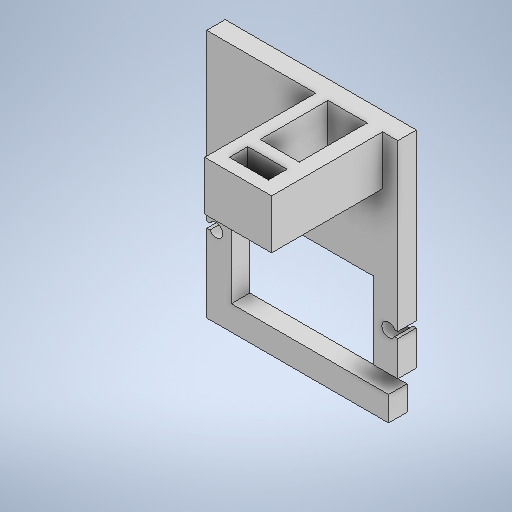
# Autodesk Inventor part: SoporteServo v2
Saved by Autodesk Inventor 2025.2 (Build 292293000, 293)
## iProperties
Created: 2025-05-14
Part Number: SoporteServo v2
Material: Generic
Document SubType Name: Modeling
Designer: cdavi
Density: 1 g/cm^3
Appearance: Default
Author: cdavi
Autodesk Inventor part; units mm, degrees
ref_plane "YZ Plane" through (0, 0, 0) normal (1, 0, 0) x (0, 1, 0)
ref_plane "XZ Plane" through (0, 0, 0) normal (0, 1, 0) x (-1, 0, 0)
ref_plane "XY Plane" through (0, 0, 0) normal (0, 0, 1) x (1, 0, 0)
sketch "Sketch1" plane through (0, 0, 0) normal (0, 0, 1) x (1, 0, 0)
  line L0 (-11.35, -6.15) -> (11.35, -6.15) construction
  line L1 (11.35, -6.15) -> (11.35, 6.15) construction
  line L2 (11.35, 6.15) -> (-11.35, 6.15) construction
  line L3 (-11.35, 6.15) -> (-11.35, -6.15) construction
  line L4 (-11.35, -6.15) -> (11.35, 6.15) construction
  line L5 (11.35, -6.15) -> (-11.35, 6.15) construction
  line L6 (-11.5, -6.3) -> (11.5, -6.3)
  line L7 (11.5, -6.3) -> (11.5, 6.3)
  line L8 (11.5, 6.3) -> (-11.5, 6.3)
  line L9 (-11.5, 6.3) -> (-11.5, -6.3)
  line L10 (-11.5, -6.3) -> (11.5, 6.3) construction
  line L11 (11.5, -6.3) -> (-11.5, 6.3) construction
  line L12 (-15.5, -13.1) -> (-15.5, 27.3)
  line L13 (-15.5, 27.3) -> (15.5, 27.3)
  line L14 (15.5, 27.3) -> (15.5, -6.15)
  line L15 (11.5, -6.15) -> (15.5, -6.15)
  line L16 (-11.5, -6.3) -> (-11.5, -9.1)
  line L17 (-11.5, -9.1) -> (14, -9.1)
  line L18 (14, -9.1) -> (14, -13.1)
  line L19 (14, -13.1) -> (-15.5, -13.1)
  circle A0 centre (-14, 0) radius 1.1
  line L20 (-14.9798, 0.5) -> (-15.5, 0.5)
  line L21 (-14.9798, -0.5) -> (-15.5, -0.5)
  line L22 (0, 0) -> (0, 6.3) construction
  circle A1 centre (14, 0) radius 1.1
  line L23 (14.9798, 0.5) -> (15.5, 0.5)
  line L24 (14.9798, -0.5) -> (15.5, -0.5)
  point P0 (15.5, -0.5)
  point P1 (15.5, 0.5)
  point P2 (14, -11.1)
  dimension "d0" = 22.7
  dimension "d1" = 12.3
  dimension "d2" = 0.15
  dimension "d3" = 0.15
  dimension "d5" = 2.95
  dimension "d6" = 4
  dimension "d7" = 21
  dimension "d8" = 4
  dimension "d9" = 4
  dimension "d13" = 2.2
  dimension "d14" = 14
  dimension "d15" = 1
  constraints: 50 end point, 8 perpendicular, 6 midpoint, 5 symmetric about line, 4 horizontal, 4 parallel, 4 point on circle, 3 point on line, 2 centre point, 2 horizontal alignment, 2 vertical, 2 vertical alignment, 1 other
  measures "d0" distance of L1.end L2.end
  measures "d1" distance between parallel lines of L0 L2
  measures "d2" distance between parallel lines of L8 L2
  measures "d3" distance between parallel lines of L9 L3
  measures "d5" distance from line of L16.end L0
  measures "d6" distance between parallel lines of L14 L7
  measures "d7" distance between parallel lines of L8 L13
  measures "d8" distance between parallel lines of L12 L9
  measures "d9" distance between parallel lines of L19 L17
  measures "d13" diameter of A0
  measures "d14" distance of L22.start A0.centre
  measures "d15" distance between parallel lines of L21 L20
extrude "Extrusion2" add sketch "Sketch1" along normal blind 3 contours L16 L17 L18 L19 L12 L21 A0 L20 L13 L14 L23 A1 L24 L15 L7 L8 L9
sketch "Sketch2" plane through (0, 0, 3) normal (0, 0, 1) x (1, 0, 0)
  line L0 (15.5, 27.3) -> (-15.5, 27.3) projected
  line L1 (-11.5, 6.3) -> (11.5, 6.3) projected
  line L2 (10.525, 27.3) -> (13.025, 27.3)
  line L3 (13.025, 27.3) -> (13.025, 19.3)
  line L4 (13.025, 19.3) -> (10.525, 19.3)
  line L5 (10.525, 19.3) -> (10.525, 27.3)
  line L6 (11.5, 6.3) -> (11.5, -6.15) projected
  line L7 (2.175, 27.3) -> (4.175, 27.3)
  line L8 (4.175, 27.3) -> (4.175, 19.3)
  line L9 (4.175, 19.3) -> (2.175, 19.3)
  line L10 (2.175, 19.3) -> (2.175, 27.3)
  line L11 (14, -9.1) -> (-11.5, -9.1) projected
  line L12 (-15.5, -13.1) -> (14, -13.1) projected
  line L13 (10.525, -9.1) -> (13.025, -9.1)
  line L14 (13.025, -9.1) -> (13.025, -13.1)
  line L15 (13.025, -13.1) -> (10.525, -13.1)
  line L16 (10.525, -13.1) -> (10.525, -9.1)
  line L17 (4.175, -9.1) -> (2.175, -9.1)
  line L18 (2.175, -9.1) -> (2.175, -13.1)
  line L19 (2.175, -13.1) -> (4.175, -13.1)
  line L20 (4.175, -13.1) -> (4.175, -9.1)
  point P0 (0, 0)
  point P1 (7.65, 6.55)
  point P2 (7.65, 6.55)
  point P3 (-1.7, 6.55)
  point P4 (10.525, -13.1)
  point P5 (4.175, -13.1)
  point P6 (2.175, -9.1)
  point P7 (10.525, -13.1)
  dimension "d19" = 2.5
  dimension "d22" = 0.975
  dimension "d23" = 2
  dimension "d24" = 6.35
  dimension "d25" = 13
  constraints: 32 end point, 8 parallel, 6 point on line, 5 collinear, 4 horizontal, 4 perpendicular
  measures "d19" distance between parallel lines of L3 L5
  measures "d22" distance between parallel lines of L5 L6
  measures "d23" distance between parallel lines of L8 L10
  measures "d24" distance between parallel lines of L5 L8
  measures "d25" distance between parallel lines of L1 L9
extrude "Extrusion3" add sketch "Sketch2" along normal blind 13.4 contours L3 L4 L5 L0 | L8 L9 L10 L0
sketch "Sketch3" plane through (-15.5, 27.3, 0) normal (0, 1, 0) x (1, 0, 0)
  line L0 (19.675, -3) -> (19.675, -16.4) projected
  line L1 (26.025, -3) -> (26.025, -16.4) projected
  line L2 (28.525, -16.4) -> (26.025, -16.4) projected
  line L3 (17.675, -16.4) -> (19.675, -16.4) projected
  line L4 (19.675, -16.4) -> (19.675, -19)
  line L5 (19.675, -19) -> (26.025, -19)
  line L6 (26.025, -19) -> (26.025, -16.4)
  line L7 (26.025, -3) -> (19.675, -3) projected
  line L8 (17.675, -16.4) -> (17.675, -21)
  line L9 (17.675, -21) -> (28.525, -21)
  line L10 (28.525, -21) -> (28.525, -16.4)
  line L11 (19.675, -16) -> (26.025, -16)
  line L12 (19.675, -14) -> (26.025, -14)
  point P0 (15.5, 0)
  dimension "d27" = 16
  dimension "d28" = 4.6
  dimension "d31" = 3
  dimension "d32" = 2
  constraints: 16 end point, 7 perpendicular, 4 point on line, 1 vertical
  measures "d27" distance between parallel lines of L5 L7
  measures "d28" distance of L3.start L8.end
  measures "d31" distance between parallel lines of L11 L5
  measures "d32" distance between parallel lines of L11 L12
extrude "Extrusion4" add sketch "Sketch3" against normal blind 8 contours L12 L1 L11 L0 | L4 L5 L6 L2 L10 L9 L8 L3
equation "\"d2\" = toleranciaServo + margenServo"
equation "\"d3\" = toleranciaServo + margenServo"
equation "\"d5\" = espesorAcrilico + margenAcrilico"
equation "\"d16\" = espesorPieza"
equation "\"d24\" = juegoCremallera + anchoCremallera - toleranciaAcrilico"
equation "\"toleranciaServo\" = 0.1"
equation "\"espesorAcrilico\" = 2.55"
equation "\"margenAcrilico\" = 0.4"
equation "\"margenServo\" = 0.05"
equation "\"largoPatilla\" = 24"
equation "\"espesorPieza\" = 3"
equation "\"anchoCremallera\" = 6.25"
equation "\"toleranciaAcrilico\" = 0.2"
equation "\"juegoCremallera\" = 0.3"
equation "\"distCremallera\" = 1.075"
body "Solid2"
